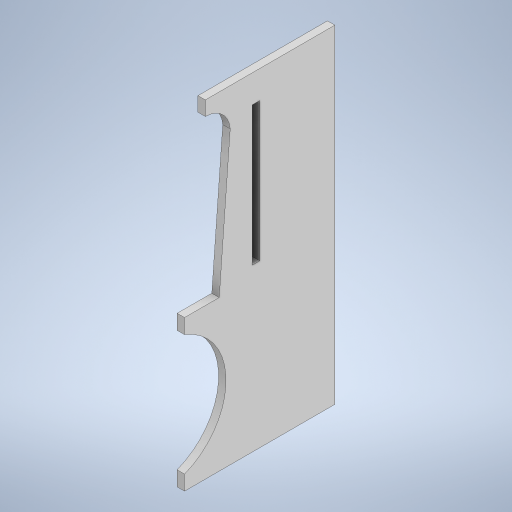
# Autodesk Inventor part: SideSupports
Saved by Autodesk Inventor 2024 (Build 280153000, 153)
## iProperties
Created: 2023-10-07
Part Number: SideSupports
Material: Generic
Document SubType Name: Modeling
Designer: chris
Density: 1 g/cm^3
Appearance: Default
Author: chris
Autodesk Inventor part; units mm, degrees
ref_plane "YZ Plane" through (0, 0, 0) normal (1, 0, 0) x (0, 1, 0)
ref_plane "XZ Plane" through (0, 0, 0) normal (0, 1, 0) x (-1, 0, 0)
ref_plane "XY Plane" through (0, 0, 0) normal (0, 0, 1) x (1, 0, 0)
sketch "Sketch1" plane through (0, 0, 0) normal (1, 0, 0) x (0, 1, 0)
  line L0 (-32.5, 13.5) -> (32.5, 13.5)
  line L1 (32.5, 13.5) -> (32.5, -13.5)
  line L2 (32.5, -13.5) -> (-32.5, -13.5)
  line L3 (-32.5, -13.5) -> (-32.5, 13.5)
  line L4 (-32.5, 13.5) -> (32.5, -13.5) construction
  line L5 (32.5, 13.5) -> (-32.5, -13.5) construction
  arc A0 (-26.1, 13.5) -> (26.1, 13.5) centre (0, 23.5) ccw
  line L6 (32.5, -13.5) -> (109.5, -13.5)
  line L7 (32.5, -1.5) -> (109.5, -7.5)
  line L8 (109.5, -7.5) -> (109.5, -13.5)
  line L9 (109.5, -7.5) -> (109.5, 4.5)
  line L10 (109.5, 4.5) -> (103.3, 4.5)
  arc A1 (90.1361, -5.9911) -> (103.3, 4.5) centre (92.5375, 4.5) ccw
  point P0 (0, 0)
  point P1 (0, 13.5)
  point P2 (32.5, -0.0243)
  point P3 (93.2849, -6.2365)
  dimension "d0" = 27
  dimension "d1" = 65
  dimension "d3" = 6.4
  dimension "d4" = 6.4
  dimension "d5" = 10
  dimension "d8" = 6
  dimension "d9" = 12
  dimension "d10" = 77
  dimension "d11" = 6.2
  dimension "d12" = 12
  dimension "d13" = 10.7625
  constraints: 22 end point, 6 point on line, 4 point on circle, 3 midpoint, 2 centre point, 2 horizontal, 2 parallel, 2 perpendicular, 2 vertical
  measures "d0" distance of L0.end L1.end
  measures "d1" distance of L1.end L2.end
  measures "d3" distance from line of L1 A0.end
  measures "d4" distance from line of L3 A0.start
  measures "d5" distance of point (0, 13.5) A0.centre
  measures "d8" distance of L7.end L6.end
  measures "d9" distance from line of L6 L7.start
  measures "d10" distance between parallel lines of L1 L8
  measures "d11" distance of L9.end L10.end
  measures "d12" distance of L7.end L9.end
  measures "d13" radius of A1
extrude "Extrusion1" add sketch "Sketch1" along normal blind 3.2 contours L0 A0 L1 L2 L3 | L1 L7 A1 L8 L6 | L7 A1 | L7 A1 L10 L9
sketch "Sketch2" plane through (3.2, 0, 0) normal (1, 0, 0) x (0, 0, -1)
  line L0 (13.5, -32.5) -> (13.5, 109.5) projected
  line L1 (13.5, 109.5) -> (51.5, 109.5)
  line L2 (51.5, 109.5) -> (51.5, -32.5)
  line L3 (51.5, -32.5) -> (13.5, -32.5)
  line L4 (13.5, -32.5) -> (13.5, 109.5)
  line L5 (-13.5, -32.5) -> (13.5, -32.5) projected
  point P0 (0, 0)
  dimension "d14" = 38
  constraints: 8 end point, 2 parallel, 1 collinear, 1 horizontal, 1 perpendicular
  measures "d14" distance of L0.end L1.end
extrude "Extrusion2" add sketch "Sketch2" against normal blind 3.2
sketch "Sketch3" plane through (3.2, 0, 0) normal (1, 0, 0) x (0, 0, -1)
  line L0 (1.5, 32.5) -> (-13.5, 32.5) construction
  line L1 (1.5, 32.5) -> (15.8, 32.5) construction
  line L2 (15.8, 37.5) -> (19, 37.5)
  line L3 (19, 37.5) -> (19, 97.5)
  line L4 (19, 97.5) -> (15.8, 97.5)
  line L5 (15.8, 97.5) -> (15.8, 37.5)
  line L6 (51.5, 109.5) -> (-4.5, 109.5) construction
  point P0 (0, 0)
  dimension "d17" = 14.3
  dimension "d18" = 3.2
  dimension "d19" = 60
  dimension "d21" = 12
  constraints: 10 end point, 2 horizontal, 2 parallel, 1 perpendicular, 1 vertical alignment
  measures "d17" distance of L0.start L1.end
  measures "d18" distance between parallel lines of L3 L5
  measures "d19" distance of L2.end L3.end
  measures "d21" distance between parallel lines of L6 L4
extrude "Extrusion3" cut sketch "Sketch3" against normal blind 3.2
body "Solid1"
